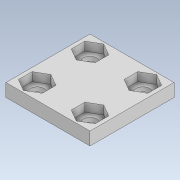
# Autodesk Inventor part: BOUCHON
Saved by Autodesk Inventor 2020 (Build 240168000, 168)
## iProperties
Created: 2020-07-10
Part Number: BOUCHON
Material: Generic
Document SubType Name: Modeling
Designer: Admin
Density: 1 g/cm^3
Appearance: Default
Author: Admin
Autodesk Inventor part; units mm, degrees
ref_plane "YZ Plane" through (0, 0, 0) normal (1, 0, 0) x (0, 1, 0)
ref_plane "XZ Plane" through (0, 0, 0) normal (0, 1, 0) x (-1, 0, 0)
ref_plane "XY Plane" through (0, 0, 0) normal (0, 0, 1) x (1, 0, 0)
sketch "Sketch1" plane through (0, 0, 0) normal (0, 1, 0) x (-1, 0, 0)
  line L0 (0, 0) -> (19.4, 0)
  line L1 (19.4, 0) -> (19.4, -19.4)
  line L2 (19.4, -19.4) -> (0, -19.4)
  line L3 (0, -19.4) -> (0, 0)
  dimension "d0" = 19.4
  dimension "d1" = 19.4
  constraints: 8 end point, 2 parallel, 1 horizontal, 1 perpendicular
  measures "d0" distance of L0.end L1.end
  measures "d1" distance of L1.end L2.end
extrude "Extrusion1" add sketch "Sketch1" along normal blind 3
sketch "Sketch2" plane through (0, 3, 0) normal (0, 1, 0) x (1, 0, 0)
  line L0 (-18.55, 2.013) -> (-18.55, 5.188)
  line L1 (-18.55, 5.188) -> (-15.8004, 6.7755)
  line L2 (-15.8004, 6.7755) -> (-13.0507, 5.188)
  line L3 (-13.0507, 5.188) -> (-13.0507, 2.013)
  line L4 (-13.0507, 2.013) -> (-15.8004, 0.4255)
  line L5 (-15.8004, 0.4255) -> (-18.55, 2.013)
  line L6 (-19.4, 0) -> (0, 0) projected
  line L7 (-19.4, 19.4) -> (-19.4, 0) projected
  dimension "d4" = 3.175
  dimension "d5" = 3.175
  dimension "d7" = 3.175
  dimension "d8" = 3.175
  dimension "d9" = 3.175
  dimension "d10" = 3.175
  dimension "d11" = 120
  dimension "d12" = 120
  dimension "d13" = 2.013
  dimension "d14" = 0.85
  constraints: 12 end point, 1 parallel, 1 vertical
  measures "d4" distance of L0.start L0.end
  measures "d5" distance of L0.end L1.end
  measures "d7" distance of L1.end L2.end
  measures "d8" distance of L2.end L3.end
  measures "d9" distance of L3.end L4.end
  measures "d10" distance of L4.end L0.start
  measures "d11" angle of L0 L5
  measures "d12" angle of L1 L0
  measures "d13" distance from line of L6 L0.start
  measures "d14" distance between parallel lines of L7 L0
extrude "Extrusion2" cut sketch "Sketch2" against normal blind 2
pattern_linear "Rectangular Pattern1" count 2 spacing 12.2 along (0, 0, -1) count 2 spacing 12.2 along (1, 0, 0) of "Extrusion2"
sketch "Sketch3" plane through (0, 1, 0) normal (0, 1, 0) x (1, 0, 0)
  circle A0 centre (-15.8, 3.6) radius 1.6
  line L0 (-19.4, 19.4) -> (-19.4, 0) projected
  line L1 (-19.4, 0) -> (0, 0) projected
  dimension "d23" = 3.2
  dimension "d24" = 3.6
  dimension "d25" = 3.6
  constraints: 1 centre point
  measures "d23" diameter of A0
  measures "d24" distance from line of L0 A0.centre
  measures "d25" distance from line of L1 A0.centre
extrude "Extrusion3" cut sketch "Sketch3" against normal through all
pattern_linear "Rectangular Pattern2" count 2 spacing 12.2 along (0, 0, -1) count 2 spacing 12.2 along (1, 0, 0) of "Extrusion3"
equation "\"d1\" = d0"
equation "\"d5\" = d4"
equation "\"d7\" = d5"
equation "\"d9\" = d7"
equation "\"d10\" = d4"
body "Solid1"
